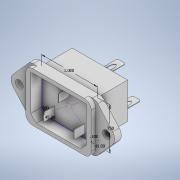
# Autodesk Inventor part: Three Pong Nema Power Insert
Saved by Autodesk Inventor 2022.1 (Build 261234000, 234)
## iProperties
Created: 2023-05-22
Part Number: Three Pong Nema Power Insert
Material: Generic
Document SubType Name: Modeling
Designer: brenden_deutschman
Density: 1 g/cm^3
Appearance: Default
Author: brenden_deutschman
Autodesk Inventor part; units mm, degrees
ref_plane "YZ Plane" through (0, 0, 0) normal (1, 0, 0) x (0, 1, 0)
ref_plane "XZ Plane" through (0, 0, 0) normal (0, 1, 0) x (-1, 0, 0)
ref_plane "XY Plane" through (0, 0, 0) normal (0, 0, 1) x (1, 0, 0)
sketch "Sketch1" plane through (0, 0, 0) normal (0, 0, 1) x (1, 0, 0)
  line L0 (-15.0495, -11.303) -> (15.0495, -11.303)
  line L1 (15.0495, -11.303) -> (15.0495, 11.303)
  line L2 (15.0495, 11.303) -> (-15.0495, 11.303)
  line L3 (-15.0495, 11.303) -> (-15.0495, -11.303)
  line L4 (-15.0495, -11.303) -> (15.0495, 11.303) construction
  line L5 (15.0495, -11.303) -> (-15.0495, 11.303) construction
  point P0 (0, 0)
  dimension "d0" = 30.099
  dimension "d1" = 22.606
  constraints: 12 end point, 2 midpoint, 2 parallel, 1 horizontal, 1 perpendicular
  measures "d0" distance of L2.end L1.end
  measures "d1" distance of L1.end L0.end
extrude "Extrusion1" add sketch "Sketch1" against normal blind 13.9954
sketch "Sketch2" plane through (0, 0, 0) normal (0, 0, 1) x (1, 0, 0)
  line L0 (-10.16, -9.525) -> (10.16, -9.525)
  line L1 (12.7, -6.985) -> (12.7, 9.525)
  line L2 (12.7, 9.525) -> (-12.7, 9.525)
  line L3 (-12.7, 9.525) -> (-12.7, -6.985)
  line L4 (-12.7, -9.525) -> (12.7, 9.525) construction
  line L5 (12.7, -9.525) -> (-12.7, 9.525) construction
  line L6 (10.16, -9.525) -> (12.7, -6.985)
  line L7 (10.16, -9.525) -> (13.7521, -9.525) construction
  line L8 (-10.16, -9.525) -> (-12.7, -6.985)
  point P0 (0, 0)
  dimension "d4" = 25.4
  dimension "d5" = 19.05
  dimension "d9" = 45
  dimension "d10" = 2.54
  dimension "d11" = 45
  dimension "d12" = 2.54
  constraints: 18 end point, 2 horizontal, 2 midpoint, 2 parallel, 1 equal length, 1 perpendicular
  measures "d4" distance of L2.end L1.end
  measures "d5" distance of L1.end L5.start
  measures "d9" angle of L0 L6
  measures "d10" horizontal distance of L0.end L1.start
  measures "d11" angle of L0 L8
  measures "d12" horizontal distance of L3.end L0.start
extrude "Extrusion2" cut sketch "Sketch2" against normal blind 0.0003
sketch "Sketch3" plane through (0, 0, 0) normal (0, 0, 1) x (1, 0, 0)
  circle A0 centre (-19.9898, 0) radius 1.7526
  circle A1 centre (19.9898, 0) radius 1.7526
  arc A2 (-22.8389, 2.5296) -> (-22.8389, -2.5296) centre (-19.9898, 0) ccw
  arc A3 (22.8389, -2.5296) -> (22.8389, 2.5296) centre (19.9898, 0) ccw
  line L0 (-15.0495, 11.303) -> (-22.8389, 2.5296)
  line L1 (-15.0495, -11.303) -> (-22.8389, -2.5296)
  line L2 (15.0495, -11.303) -> (22.8389, -2.5296)
  line L3 (15.0495, 11.303) -> (15.0495, -11.303) projected
  line L4 (-15.0495, 11.303) -> (15.0495, 11.303)
  line L5 (15.0495, 11.303) -> (22.8389, 2.5296)
  line L6 (15.0495, 11.303) -> (-15.0495, 11.303) projected
  line L7 (-15.0495, 11.303) -> (15.0495, 11.303)
  line L8 (-15.0495, -11.303) -> (15.0495, -11.303) projected
  line L9 (-15.0495, -11.303) -> (15.0495, -11.303)
  line L10 (-15.0495, 11.303) -> (-15.0495, -11.303) projected
  line L11 (-15.0495, 11.303) -> (-15.0495, -11.303)
  line L12 (-12.7, -6.985) -> (-12.7, 9.525) projected
  line L13 (-12.7, 9.525) -> (12.7, 9.525) projected
  line L14 (-12.7, 9.525) -> (12.7, 9.525)
  line L15 (12.7, 9.525) -> (12.7, -6.985) projected
  line L16 (12.7, 9.525) -> (12.7, -6.985)
  line L17 (12.7, -6.985) -> (10.16, -9.525) projected
  line L18 (12.7, -6.985) -> (10.16, -9.525)
  line L19 (10.16, -9.525) -> (-10.16, -9.525) projected
  line L20 (10.16, -9.525) -> (-10.16, -9.525)
  line L21 (-10.16, -9.525) -> (-12.7, -6.985) projected
  line L22 (-10.16, -9.525) -> (-12.7, -6.985)
  line L23 (-12.7, -6.985) -> (-12.7, 9.525)
  point P0 (0, 0)
  point P1 (-20.0025, 0)
  dimension "d17" = 3.5052
  dimension "d19" = 7.62
  dimension "d20" = 7.62
  dimension "d21" = 7.7894
  dimension "d24" = 20.0025
  constraints: 28 end point, 4 centre point, 4 collinear, 4 point on circle, 4 tangent, 3 horizontal, 2 coincident, 1 parallel, 1 perpendicular, 1 vertical
  measures "d17" diameter of A0
  measures "d19" diameter of A2
  measures "d20" diameter of A3
  measures "d21" horizontal distance of L1.start L1.end
  measures "d24" distance of point (0, 0) point (-20.002, 0)
extrude "Extrusion3" add sketch "Sketch3" along normal blind 2.9972 contours L0 L10 L1 A2 | L5 A3 L2 L3
extrude "Extrusion4" add sketch "Sketch3" along normal blind 5.0038 contours L4 L3 L8 L10
sketch "Sketch4" plane through (0, 0, -13.9954) normal (0, 0, -1) x (-1, 0, 0)
  line L0 (-12.7, 9.525) -> (-12.7, -6.985) projected
  line L1 (12.7, 9.525) -> (-12.7, 9.525) projected
  line L2 (-12.7, 9.525) -> (12.7, 9.525)
  line L3 (12.7, -6.985) -> (12.7, 9.525) projected
  line L4 (12.7, 9.525) -> (12.7, -6.985)
  line L5 (10.16, -9.525) -> (12.7, -6.985) projected
  line L6 (12.7, -6.985) -> (10.16, -9.525)
  line L7 (-10.16, -9.525) -> (10.16, -9.525) projected
  line L8 (10.16, -9.525) -> (-10.16, -9.525)
  line L9 (-12.7, -6.985) -> (-10.16, -9.525) projected
  line L10 (-10.16, -9.525) -> (-12.7, -6.985)
  line L11 (-12.7, -6.985) -> (-12.7, 9.525)
  line L12 (-15.0495, 11.303) -> (15.0495, 11.303) projected
  line L13 (15.0495, -11.303) -> (-15.0495, -11.303) projected
  line L14 (-15.0495, 11.303) -> (-15.0495, -11.303)
  line L15 (-15.0495, -11.303) -> (15.0495, -11.303)
  line L16 (15.0495, 11.303) -> (15.0495, -11.303) projected
  line L17 (15.0495, -11.303) -> (15.0495, 11.303)
  line L18 (-15.0495, 11.303) -> (-15.0495, -11.303) projected
  line L19 (15.0495, 11.303) -> (-15.0495, 11.303)
  point P0 (0, 0)
  constraints: 20 end point, 5 equal length, 3 perpendicular, 1 horizontal, 1 vertical
extrude "Extrusion5" cut sketch "Sketch4" against normal blind 13.9954
sketch "Sketch5" plane through (0, 0, -13.9954) normal (0, 0, -1) x (-1, 0, 0)
  circle A0 centre (0, 3.81) radius 0.9525
  line L0 (-10.16, -9.525) -> (10.16, -9.525) projected
  circle A1 centre (-6.985, -3.81) radius 0.9525
  circle A2 centre (6.985, -3.81) radius 0.9525
  line L1 (-6.985, -3.81) -> (-6.985, -5.715)
  line L2 (-6.985, -5.715) -> (-8.89, -5.715)
  line L3 (-8.89, -5.715) -> (-8.89, -3.175)
  line L4 (-6.985, -5.715) -> (-5.0675, -5.715)
  line L5 (-5.0675, -5.715) -> (-5.0675, -3.175)
  line L6 (-8.89, -3.175) -> (-8.0476, -1.905)
  line L7 (-5.0675, -3.175) -> (-5.9099, -1.905)
  line L8 (-5.9099, -1.905) -> (-8.0476, -1.905)
  line L9 (6.985, -3.81) -> (6.985, -5.715)
  line L10 (6.985, -5.715) -> (5.08, -5.715)
  line L11 (5.08, -5.715) -> (5.08, -3.175)
  line L12 (5.08, -3.175) -> (6.0325, -1.9853)
  line L13 (6.985, -5.715) -> (8.89, -5.715)
  line L14 (8.89, -5.715) -> (8.89, -3.175)
  line L15 (8.89, -3.175) -> (7.9375, -1.9853)
  line L16 (7.9375, -1.9853) -> (6.0325, -1.9853)
  line L17 (0, 3.81) -> (0, 5.7246)
  line L18 (0, 5.7246) -> (-1.905, 5.7246)
  line L19 (-1.905, 5.7246) -> (-1.905, 3.1846)
  line L20 (0, 5.7246) -> (1.905, 5.7246)
  line L21 (1.905, 5.7246) -> (1.905, 3.1846)
  line L22 (1.905, 3.1846) -> (0.9525, 1.995)
  line L23 (0.9525, 1.995) -> (-0.9525, 1.995)
  line L24 (-0.9525, 1.995) -> (-1.905, 3.1846)
  point P0 (0, 0)
  dimension "d32" = 1.905
  dimension "d36" = 1.905
  dimension "d37" = 1.905
  dimension "d38" = 1.905
  dimension "d39" = 1.905
  dimension "d40" = 2.54
  dimension "d41" = 1.524
  dimension "d42" = 146.443
  dimension "d43" = 1.524
  dimension "d44" = 1.905
  dimension "d45" = 1.524
  dimension "d46" = 1.905
  dimension "d47" = 1.524
  dimension "d48" = 1.905
  dimension "d49" = 2.54
  dimension "d50" = 1.905
  dimension "d51" = 1.524
  constraints: 48 end point, 7 perpendicular, 4 horizontal, 3 centre point, 3 vertical, 2 parallel
  measures "d32" diameter of A0
  measures "d36" diameter of A1
  measures "d37" diameter of A2
  measures "d38" distance of L1.start L1.end
  measures "d39" distance of L1.end L2.end
  measures "d40" distance of L2.end L3.end
  measures "d41" distance of L3.end L6.end
  measures "d42" angle of L6 L3
  measures "d43" distance of L5.end L7.end
  measures "d44" distance of L9.end L10.end
  measures "d45" distance of L11.end L12.end
  measures "d46" distance of L9.end L13.end
  measures "d47" distance of L14.end L15.end
  measures "d48" distance of L17.end L18.end
  measures "d49" distance of L18.end L19.end
  measures "d50" distance of L17.end L20.end
  measures "d51" distance of L21.end L22.end
extrude "Extrusion6" add sketch "Sketch5" along normal blind 0.127 contours A0 | L20 L21 L22 L23 L24 L19 L18 | A1 | L2 L3 L6 L8 L7 L5 L4 | A2 | L10 L11 L12 L16 L15 L14 L13
sketch "Sketch6" plane through (0, 0, -14.1224) normal (0, 0, -1) x (-1, 0, 0)
  line L0 (-1.905, 5.7246) -> (1.905, 5.7246) projected
  line L1 (-1.905, 5.7246) -> (1.905, 5.7246)
  line L2 (1.905, 5.7246) -> (1.905, 5.4706)
  line L3 (1.905, 5.7246) -> (1.905, 3.1846) projected
  line L4 (1.905, 5.4706) -> (-1.905, 5.4706)
  line L5 (-1.905, 5.7246) -> (-1.905, 3.1846) projected
  line L6 (-8.89, -5.715) -> (-5.0675, -5.715) projected
  line L7 (-8.89, -5.715) -> (-5.0675, -5.715)
  line L8 (-5.0675, -5.715) -> (-5.0675, -5.461)
  line L9 (-5.0675, -5.715) -> (-5.0675, -3.175) projected
  line L10 (-5.0675, -5.461) -> (-8.89, -5.461)
  line L11 (-8.89, -5.715) -> (-8.89, -3.175) projected
  line L12 (-8.89, -5.715) -> (-5.0675, -5.715)
  line L13 (5.08, -5.715) -> (8.89, -5.715) projected
  line L14 (8.89, -5.715) -> (8.89, -3.175) projected
  line L15 (5.08, -5.715) -> (8.89, -5.715)
  line L16 (8.89, -5.715) -> (8.89, -5.461)
  line L17 (8.89, -5.461) -> (5.08, -5.461)
  line L18 (5.08, -3.175) -> (5.08, -5.715) projected
  point P0 (0, 0)
  dimension "d54" = 0.254
  dimension "d55" = 0.254
  dimension "d56" = 0.254
  constraints: 20 end point, 5 point on line, 4 perpendicular, 2 equal length, 2 horizontal
  measures "d54" distance of L0.end L2.end
  measures "d55" distance of L6.end L8.end
  measures "d56" distance of L13.end L16.end
extrude "Extrusion7" add sketch "Sketch6" along normal blind 9.7536
sketch "Sketch7" plane through (5.0675, -5.461, -14.1224) normal (0, 1, 0) x (1, 0, 0)
  line L0 (0, -0.127) -> (0, 9.7536) projected
  ellipse E0 centre (1.9175, 4.8133) end of major axis (1.9175, 2.3495) minor radius 0.9906
  line L1 (-3.1625, -0.127) -> (-3.1625, 9.7536) projected
  line L2 (-3.1625, 4.8133) -> (-5.0675, 4.8133)
  ellipse E1 centre (-5.0675, 4.8133) end of major axis (-5.0675, 2.3495) minor radius 0.9906
  ellipse E2 centre (-12.0525, 4.8133) end of major axis (-12.0525, 2.3495) minor radius 0.9906
  line L3 (-13.9575, -0.127) -> (-10.1475, -0.127) projected
  line L4 (3.8225, 0) -> (3.8225, 9.7536) projected
  line L5 (-10.1475, 0) -> (-10.1475, 9.7536) projected
  line L6 (0, 9.7536) -> (3.8225, 9.7536) projected
  line L7 (-13.9575, 9.7536) -> (-10.1475, 9.7536) projected
  point P0 (-5.0675, -14.1224)
  point P1 (-10.1475, 4.8768)
  dimension "d61" = 2.4638
  dimension "d62" = 2.4638
  dimension "d63" = 0.9906
  dimension "d64" = 0.9906
  dimension "d59" = 2.4638
  dimension "d60" = 0.9906
  dimension "d65" = 1.905
  dimension "d66" = 1.905
  dimension "d67" = 1.905
  dimension "d68" = 4.9403
  dimension "d69" = 4.9403
  constraints: 3 horizontal, 2 end point, 2 midpoint, 1 centre point, 1 coincident, 5 other
  measures "d65" distance from line of L4 E0.centre
  measures "d66" distance from line of L1 L2.end
  measures "d67" horizontal distance of point (-10.148, 4.877) point (-12.053, 4.813)
  measures "d68" distance from line of L6 E0.centre
  measures "d69" distance from line of L7 point (-12.053, 4.813)
extrude "Extrusion8" cut sketch "Sketch7" along normal through all both and the other way through all
sketch "Sketch8" plane through (0, 0, -0.0003) normal (0, 0, 1) x (1, 0, 0)
  line L0 (1.905, 5.7246) -> (-1.905, 5.7246) projected
  line L1 (1.905, 5.4706) -> (-1.905, 5.4706) projected
  line L2 (-1.905, 5.4706) -> (-1.905, 5.7246) projected
  line L3 (-1.905, 5.5976) -> (0, 5.5976)
  line L4 (0.127, 3.6926) -> (0.127, 7.5026)
  line L5 (0.127, 7.5026) -> (-0.127, 7.5026)
  line L6 (-0.127, 7.5026) -> (-0.127, 3.6926)
  line L7 (-0.127, 3.6926) -> (0.127, 3.6926)
  line L8 (8.89, -5.715) -> (5.0675, -5.715) projected
  line L9 (6.8518, -7.493) -> (7.1058, -7.493)
  line L10 (7.1058, -7.493) -> (7.1058, -3.683)
  line L11 (7.1058, -7.493) -> (10.9158, -7.493) construction
  line L12 (7.1058, -3.683) -> (6.8518, -3.683)
  line L13 (6.8518, -3.683) -> (6.8518, -7.493)
  line L14 (-8.89, -5.715) -> (-5.08, -5.715) projected
  line L15 (-6.858, -5.588) -> (-4.953, -5.588) construction
  line L16 (-6.858, -7.493) -> (-7.112, -7.493)
  line L17 (-7.112, -7.493) -> (-7.112, -3.683)
  line L18 (-7.112, -3.683) -> (-6.858, -3.683)
  line L19 (-6.858, -3.683) -> (-6.858, -7.493)
  point P0 (0, 0)
  point P1 (6.9788, -5.715)
  point P2 (-6.985, -5.715)
  dimension "d75" = 0.254
  dimension "d79" = 90
  dimension "d80" = 3.81
  dimension "d81" = 0.254
  dimension "d82" = 3.81
  dimension "d83" = 0.254
  dimension "d84" = 0.127
  dimension "d89" = 0.254
  dimension "d90" = 3.81
  dimension "d91" = 0.254
  dimension "d92" = 0.127
  dimension "d93" = 1.778
  constraints: 30 end point, 5 perpendicular, 4 horizontal, 3 midpoint, 2 vertical
  measures "d75" distance of L4.end L5.end
  measures "d79" angle of L11 L10
  measures "d80" distance of L12.end L9.start
  measures "d81" distance of L10.end L12.end
  measures "d82" distance of L9.end L10.end
  measures "d83" distance of L9.start L9.end
  measures "d84" distance from line of point (6.979, -5.715) L13
  measures "d89" distance of L16.start L16.end
  measures "d90" distance of L18.end L16.start
  measures "d91" distance of L17.end L18.end
  measures "d92" distance from line of point (-6.985, -5.715) L19
  measures "d93" distance from line of point (-6.985, -5.715) L16
extrude "Extrusion9" add sketch "Sketch8" along normal blind 5.0038 contours L4 L1 L6 L0 | L0 L6 L5 L4 | L4 L7 L6 L1 | L10 L9 L13 L8 | L8 L13 L12 L10 | L17 L18 L19 L14 | L14 L19 L16 L17
fillet "Fillet1" radius 3.175 8 edges at (15.0495, 11.303, 4.0005) (15.0495, 11.303, 1.4986) (15.0495, -11.303, 4.0005) (-15.0495, 11.303, 4.0005) (-15.0495, 11.303, 1.4986) (-15.0495, -11.303, 4.0005) (-15.0495, -11.303, 1.4986) (15.0495, -11.303, 1.4986)
chamfer "Chamfer1" distance 0.508 angle 45 11 edges at (-6.985, -3.683, 5.0035) (0, 7.5026, 5.0035) (6.9788, -3.683, 5.0035) (-6.985, -7.493, 5.0035) (6.9788, -7.493, 5.0035) (1.905, 5.5976, -23.876) (-1.905, 5.5976, -23.876) (8.89, -5.588, -23.876) (5.0675, -5.588, -23.876) (-5.08, -5.588, -23.876) (-8.89, -5.588, -23.876)
body "Solid1"
